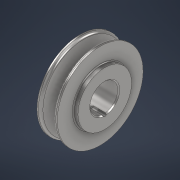
# Autodesk Inventor part: Ролик
Saved by Autodesk Inventor 2021 (Build 250183000, 183)
## iProperties
Created: 2022-05-01
Part Number: Ролик
Material: Steel, Cast
Document SubType Name: Modeling
Designer: DuctopwH
Density: 7.85 g/cm^3
Appearance: Semi-Polished
Author: DuctopwH
Autodesk Inventor part; units mm, degrees
ref_plane "YZ Plane" through (0, 0, 0) normal (1, 0, 0) x (0, 1, 0)
ref_plane "XZ Plane" through (0, 0, 0) normal (0, 1, 0) x (-1, 0, 0)
ref_plane "XY Plane" through (0, 0, 0) normal (0, 0, 1) x (1, 0, 0)
sketch "Sketch1" plane through (0, 0, 0) normal (0, 0, 1) x (1, 0, 0)
  line L0 (27.5, 0) -> (-27.5, 0)
  line L1 (0, 0) -> (0, 26) construction
  line L2 (0, 26) -> (-25.5, 26)
  line L3 (-25.5, 26) -> (-27.5, 28)
  line L4 (-27.5, 28) -> (-27.5, 50)
  line L5 (-27.5, 50) -> (-19, 50)
  line L6 (-19, 50) -> (-19, 80)
  line L7 (-19, 80) -> (-16.25, 80)
  line L8 (-11.45, 76.4) -> (-4.8, 53.6)
  line L9 (0, 26) -> (25.5, 26)
  line L10 (25.5, 26) -> (27.5, 28)
  line L11 (27.5, 28) -> (27.5, 50)
  line L12 (27.5, 50) -> (19, 50)
  line L13 (19, 50) -> (19, 80)
  line L14 (19, 80) -> (16.25, 80)
  line L15 (11.45, 76.4) -> (4.8, 53.6)
  arc A0 (-4.8, 53.6) -> (4.8, 53.6) centre (0, 55) ccw
  arc A1 (16.25, 80) -> (11.45, 76.4) centre (16.25, 75) ccw
  arc A2 (-11.45, 76.4) -> (-16.25, 80) centre (-16.25, 75) ccw
  point P0 (-12.5, 80)
  point P1 (0, 37.1429)
  point P2 (12.5, 80)
  point P3 (0, 50)
  dimension "d0" = 160
  dimension "d1" = 52
  dimension "d2" = 100
  dimension "d3" = 25
  dimension "d4" = 38
  dimension "d5" = 55
  dimension "d7" = 2
  dimension "d8" = 45
  dimension "d9" = 5
  dimension "d21" = 100
  constraints: 32 end point, 9 point on line, 7 point on circle, 6 symmetric about line, 6 tangent, 3 centre point, 3 perpendicular, 2 equal radius, 2 horizontal, 2 vertical, 1 coincident, 1 midpoint
  measures "d0" diameter of L14 L0
  measures "d1" diameter of L2 L0
  measures "d2" diameter of L5 L0
  measures "d3" distance of point (12.5, 80) point (-12.5, 80)
  measures "d4" distance between parallel lines of L13 L6
  measures "d5" distance between parallel lines of L11 L4
  measures "d7" horizontal distance of L3.end L2.end
  measures "d8" angle of L3 L4
  measures "d9" radius of A0
  measures "d21" diameter of point (0, 50) L0
revolve "Revolution1" add sketch "Sketch1" angle 360 about axis through (27.5, 0, 0) along (-1, 0, 0)
sketch "Sketch3" plane through (27.5, 0, 0) normal (1, 0, 0) x (0, 0, -1)
  line L0 (0, 0) -> (0, -26)
  circle A0 centre (0, 0) radius 26 projected
  constraints: 2 end point, 1 coincident, 1 vertical, 1 vertical alignment, 1 other
hole "Hole1" at (27.5, -26, 0) direction (-1, 0, 0) diameter 6.917 depth 25 thread size "M8x1" class "6H" standard "ANSI Metric M Profile"
fillet "Fillet1" radius 2 2 edges at (19, -50, 0) (-19, -50, 0)
body "Solid1"
